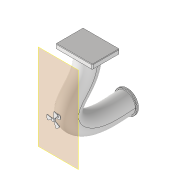
# Autodesk Inventor part: Rohr_3
Saved by Autodesk Inventor 2020 (Build 240168000, 168)
## iProperties
Created: 2020-04-08
Part Number: Rohr_3
Material: Generisch
Document SubType Name: Modeling
Designer: franz
Density: 1 g/cm^3
Appearance: Vorgabe
Author: franz
Autodesk Inventor part; units mm, degrees
ref_plane "YZ Plane" through (0, 0, 0) normal (1, 0, 0) x (0, 1, 0)
ref_plane "XZ Plane" through (0, 0, 0) normal (0, 1, 0) x (-1, 0, 0)
sketch "Skizze1" plane through (0, 0, 0) normal (0, 0, 1) x (1, 0, 0)
  circle A0 centre (0, 0) radius 100
  circle A1 centre (0, 0) radius 110
  dimension "d0" = 200
  dimension "d1" = 220
  constraints: 2 centre point, 2 coincident
  measures "d0" diameter of A0
  measures "d1" diameter of A1
sketch "Skizze2" plane through (0, 0, 0) normal (1, 0, 0) x (0, 1, 0)
  spline S0 degree 4 poles (0, 0) (0, 122.8381) (-94.2197, 545.0613) (335.1522, 848.2344) (389.0665, 412.2576) (673.9491, 412.2576) knots 0 0 0 0 0 0.50007 1 1 1 1 1
  line L0 (0, -89.8006) -> (0, 89.8006) construction
  arc A0 (-5.918, -70.8449) -> (-5.918, 70.8449) centre (-427.0049, 0) ccw construction
  line L1 (475.0993, 412.2576) -> (872.7989, 412.2576) construction
  arc A1 (522.456, 435.9353) -> (825.4422, 435.9353) centre (673.9491, 908.7332) ccw construction
  point P0 (44.2776, 469.5557)
  point P1 (250.8284, 618.9754)
  constraints: 4 end point, 4 midpoint, 2 centre point, 2 horizontal, 2 point on circle, 2 vertical, 6 other
sweep "Sweeping1" add profiles "Skizze1" path "Skizze2"
sketch "Skizze3" plane through (0, 673.9491, 412.2576) normal (0, 1, 0) x (1, 0, 0)
  circle A0 centre (0, 0) radius 131.4329
  point P0 (0, 412.2576)
  constraints: 1 centre point
extrude "Extrusion1" add sketch "Skizze3" along normal blind 10
sketch "Skizze4" plane through (0, 683.9491, 412.2576) normal (0, 1, 0) x (1, 0, 0)
  line L0 (200, 150) -> (-200, 150)
  line L1 (-200, 150) -> (-200, -150)
  line L2 (-200, -150) -> (200, -150)
  line L3 (200, -150) -> (200, 150)
  line L4 (200, 150) -> (-200, -150) construction
  line L5 (-200, 150) -> (200, -150) construction
  point P0 (0, 412.2576)
  point P1 (0, 0)
  dimension "d6" = 400
  dimension "d7" = 300
  constraints: 12 end point, 2 midpoint, 2 parallel, 1 horizontal, 1 perpendicular
  measures "d6" distance of L2.end L1.end
  measures "d7" distance of L1.end L0.end
extrude "Extrusion2" add sketch "Skizze4" along normal blind 50
chamfer "Fase1" distance 5 angle 45 8 edges at (0, 683.9491, 562.2576) (-200, 683.9491, 412.2576) (0, 683.9491, 262.2576) (200, 683.9491, 412.2576) (200, 733.9491, 412.2576) (0, 733.9491, 262.2576) (0, 733.9491, 562.2576) (-200, 733.9491, 412.2576)
chamfer "Fase2" distance 10 angle 45 4 edges at (-200, 708.9491, 562.2576) (200, 708.9491, 562.2576) (200, 708.9491, 262.2576) (-200, 708.9491, 262.2576)
fillet "Rundung1" radius 2 3 edges at (-131.4329, 673.9491, 412.2576) (-131.4329, 683.9491, 412.2576) (-110, 673.9491, 412.2576)
ref_plane "Arbeitsebene1" through (0.0061, 227.4141, 731.2767) normal (0, 0, 1) x (1, 0, 0)
sketch "Skizze5" plane through (0.0061, 227.4141, 731.2767) normal (0, 0, 1) x (1, 0, 0)
  circle A0 centre (0, 0) radius 25
  point P0 (-0.0061, -227.4141)
  dimension "d17" = 50
  constraints: 1 centre point
  measures "d17" diameter of A0
extrude "Extrusion3" add sketch "Skizze5" against normal mid plane 4.769
sketch "Skizze6" plane through (0.0061, 227.4141, 733.6612) normal (0, 0, 1) x (1, 0, 0)
  circle A0 centre (0, 0) radius 7.5
  point P0 (-0.0061, -227.4141)
  dimension "d20" = 15
  constraints: 1 centre point
  measures "d20" diameter of A0
extrude "Extrusion4" add sketch "Skizze6" along normal blind 40
sketch "Skizze7" plane through (0.0061, 227.4141, 773.6612) normal (0, 0, 1) x (1, 0, 0)
  circle A0 centre (0, 0) radius 15
  point P0 (-0.0061, -227.4141)
  dimension "d23" = 30
  constraints: 1 centre point
  measures "d23" diameter of A0
extrude "Extrusion5" add sketch "Skizze7" along normal blind 20
sketch "Skizze8" plane through (0, 0, 0) normal (1, 0, 0) x (0, 1, 0)
  line L0 (242.4141, 773.6612) -> (242.4141, 793.6612) projected
  line L1 (242.4141, 783.6612) -> (302.4141, 783.6612)
  line L2 (302.4141, 783.6612) -> (302.4141, 778.6612)
  line L3 (302.4141, 778.6612) -> (242.4141, 778.6612)
  line L4 (242.4141, 778.6612) -> (242.4141, 783.6612)
  line L5 (242.4141, 773.6612) -> (212.4141, 773.6612) projected
  line L6 (227.4141, 808.0108) -> (227.4141, 746.0125)
  point P0 (0, 0)
  dimension "d26" = 60
  dimension "d27" = 5
  dimension "d28" = 5
  constraints: 10 end point, 2 parallel, 2 vertical, 1 horizontal, 1 midpoint, 1 perpendicular
  measures "d26" distance of L2.end L3.end
  measures "d27" distance of L1.end L2.end
  measures "d28" distance between parallel lines of L5 L3
revolve "Umdrehung1" add sketch "Skizze8" angle 40 about axis through (0, 227.4141, 808.0108) along (0, 0, -1)
fillet "Rundung2" radius 5 4 edges at (48.2091, 284.8675, 781.1612) (9.6443, 238.9078, 781.1612) (0, 302.4141, 781.1612) (0, 242.4141, 781.1612)
pattern_circular "Runde Anordnung1" count 3 over 360 about axis through (0.0061, 227.4141, 773.6612) along (0, 0, 1) of "Umdrehung1", "Rundung2"
sketch "Skizze9" plane through (0, 0, 0) normal (0, 0, -1) x (-1, 0, 0)
  circle A0 centre (0, 0) radius 125
  circle A1 centre (0, 0) radius 100 projected
  point P0 (-100, 0)
  dimension "d34" = 250
  constraints: 1 centre point, 1 coincident, 1 horizontal alignment
  measures "d34" diameter of A0
extrude "Extrusion6" add sketch "Skizze9" along normal blind 20
chamfer "Fase3" distance 4 angle 45 4 edges at (125, 0, 0) (-110, 0, 0) (125, 0, -20) (100, 0, -20)
